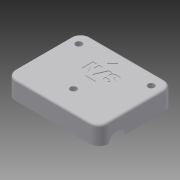
# Autodesk Inventor part: 137 V Dipole Top
Saved by Autodesk Inventor 2014 (Build 180170000, 170)
## iProperties
Created: 2023-07-11
Part Number: 137 V Dipole Top
Material: Generic
Document SubType Name: Modeling
Designer: VMUser
Density: 1 g/cm^3
Appearance: Default
Author: VMUser
Autodesk Inventor part; units mm, degrees
ref_plane "YZ Plane" through (0, 0, 0) normal (1, 0, 0) x (0, 1, 0)
sketch "Sketch1" plane through (0, 0, 0) normal (0, 1, 0) x (-1, 0, 0)
  line L0 (0, 0) -> (63.5, 0)
  line L1 (63.5, 0) -> (63.5, -50.8)
  line L2 (63.5, -50.8) -> (0, -50.8)
  line L3 (0, -50.8) -> (0, 0)
  line L4 (31.75, -50.8) -> (31.75, -30.48)
  line L5 (31.75, -30.48) -> (63.5, -12.1491)
  line L6 (31.75, -30.48) -> (0, -12.1491)
  line L7 (31.75, -30.48) -> (68.4117, -30.48) construction
  dimension "d0" = 63.5
  dimension "d1" = 50.8
  dimension "d2" = 20.32
  dimension "d3" = 120
  dimension "d4" = 150
  dimension "d5" = 120
  constraints: 16 end point, 3 parallel, 2 horizontal, 2 point on line, 1 equal length, 1 midpoint, 1 perpendicular
  measures "d0" distance of L1.end L2.end
  measures "d1" distance of L0.end L1.end
  measures "d2" distance of L4.start L4.end
  measures "d3" angle of L4 L5
  measures "d4" angle of L7 L6
  measures "d5" angle of L5 L6
extrude "Extrusion1" add sketch "Sketch1" along normal blind 12.7
ref_plane "Work Plane1" through (0, 0, 0) normal (0.8660254, 0, 0.5) x (0, 1, 0)
ref_plane "Work Plane2" through (-31.75, 0, -50.8) normal (-1, 0, 0) x (0, 0, 1)
sketch "Sketch2" plane through (0, 0, 0) normal (0.8660254, 0, 0.5) x (0, 1, 0)
  circle A0 centre (0, -10.5215) radius 4.826
  point P0 (0, 0)
  point P1 (0, -10.5215)
  dimension "d10" = 9.652
  constraints: 1 centre point, 1 coincident
  measures "d10" diameter of A0
extrude "Extrusion2" cut sketch "Sketch2" against normal up to surface surface through (-31.75, 0, -50.8) normal (-1, 0, 0)
mirror "Mirror2" about plane through (-31.75, 0, -50.8) normal (-1, 0, 0) of "Extrusion2"
sketch "Sketch5" plane through (0, 0, -50.8) normal (0, 0, -1) x (-1, 0, 0)
  circle A0 centre (31.75, 0) radius 3.556
  dimension "d18" = 7.112
  constraints: 1 centre point, 1 coincident
  measures "d18" diameter of A0
extrude "Extrusion4" cut sketch "Sketch5" against normal blind 20.32
sketch "Sketch6" plane through (0, 0, 0) normal (0, -1, 0) x (1, 0, 0)
  line L0 (-35.306, -33.9995) -> (-63.5, -17.7217) projected
  circle A0 centre (-60.2004, -19.6267) radius 1.3335
  line L1 (14.7857, -57.3474) -> (-82.6851, -1.0726) projected
  point P0 (0, 0)
  dimension "d21" = 2.667
  dimension "d23" = 1.905
  constraints: 1 centre point, 1 point on line
  measures "d21" diameter of A0
  measures "d23" vertical distance of L0.end A0.centre
revolve "Revolution1" cut sketch "Sketch6" angle 360 about axis through (-68.7607, 0, -9.1118) along (-0.8660254, 0, 0.5)
mirror "Mirror3" about plane through (-31.75, 0, -50.8) normal (-1, 0, 0) of "Revolution1"
sketch "Sketch11" plane through (0, 0, 0) normal (0, -1, 0) x (1, 0, 0)
  line L0 (-35.306, -50.8) -> (-35.306, -33.9995) projected
  circle A0 centre (-35.306, -42.3998) radius 1.016
  line L1 (-31.75, -60.96) -> (-31.75, 10.16) projected
  point P0 (0, 0)
  dimension "d33" = 2.032
  constraints: 1 centre point, 1 midpoint
  measures "d33" diameter of A0
revolve "Revolution4" cut sketch "Sketch11" angle 360 about axis through (-31.75, 0, -50.8) along (0, 0, 1)
sketch "Sketch12" plane through (0, 0, 0) normal (0, -1, 0) x (1, 0, 0)
  arc A0 (-6.9707, -10.6011) -> (-9.2804, -11.9346) centre (-8.1256, -11.2678) ccw projected
  arc A1 (-54.2196, -11.9346) -> (-56.5293, -10.6011) centre (-55.3744, -11.2678) ccw projected
  arc A2 (-9.3141, -10.6632) -> (-54.1859, -10.6632) centre (-31.75, -56.2403) ccw
  arc A3 (-9.4587, -11.3001) -> (-54.0413, -11.3001) centre (-31.75, -56.2403) ccw
  arc A4 (-8.881, -10.169) -> (-54.619, -10.169) centre (-31.75, -56.2403) ccw
  dimension "d35" = 50.8
  dimension "d36" = 0.635
  dimension "d37" = 0.635
  constraints: 12 point on circle, 3 centre point
  measures "d35" radius of A2
  measures "d36" radial gap between concentric circles of A4 A2
  measures "d37" radial gap between concentric circles of A2 A3
extrude "Extrusion5" cut sketch "Sketch12" against normal blind 1.27
sketch "Sketch13" plane through (0, 0, 0) normal (0, -1, 0) x (1, 0, 0)
  arc A0 (-35.306, -41.3838) -> (-35.306, -43.4158) centre (-35.306, -42.3998) ccw projected
  arc A1 (-61.3553, -18.96) -> (-59.0456, -20.2935) centre (-60.2004, -19.6267) ccw projected
  arc A2 (-59.8182, -20.9043) -> (-36.3024, -42.2011) centre (-29.5982, -11.167) ccw
  arc A3 (-60.4761, -20.9314) -> (-36.2063, -42.8707) centre (-29.5982, -11.167) ccw
  arc A4 (-59.2583, -20.5704) -> (-35.9624, -41.6242) centre (-29.5982, -11.167) ccw
  point P0 (0, 0)
  dimension "d40" = 31.75
  dimension "d41" = 0.635
  dimension "d42" = 0.635
  constraints: 12 point on circle, 3 centre point
  measures "d40" radius of A2
  measures "d41" radial gap between concentric circles of A4 A2
  measures "d42" radial gap between concentric circles of A2 A3
extrude "Extrusion6" cut sketch "Sketch13" against normal blind 1.27
mirror "Mirror4" about plane through (-31.75, 0, -50.8) normal (-1, 0, 0) of "Extrusion6"
sketch "Sketch14" plane through (0, 0, 0) normal (0, -1, 0) x (1, 0, 0)
  arc A0 (-35.9624, -41.6242) -> (-36.2063, -42.8707) centre (-35.306, -42.3998) ccw projected
  arc A1 (-27.2937, -42.8707) -> (-27.5376, -41.6242) centre (-28.194, -42.3998) ccw projected
  line L0 (-35.306, -42.3998) -> (-56.388, -42.3998) construction
  line L1 (-31.75, -34.2474) -> (-31.75, -30.48) construction
  point P0 (-31.75, -24.9074)
  point P1 (0, 0)
  point P2 (-31.75, -14.1124)
  point P3 (-7.112, -42.3998)
  dimension "d45" = 10.795
  dimension "d46" = 21.082
  constraints: 2 end point, 1 coincident, 1 horizontal, 1 symmetric about line
  measures "d45" distance of point (-31.75, -24.907) point (-31.75, -14.112)
  measures "d46" distance of L0.start L0.end
hole "Hole1" at (-31.75, 0, -14.1124) at (-56.388, 0, -42.3998) at (-7.112, 0, -42.3998) direction (0, 1, 0) diameter 4.3942 end through all counterbore diameter 10.287 counterbore depth 6.35
fillet "Fillet1" radius 6.35 4 edges at (-63.5, 6.35, -50.8) (0, 6.35, -50.8) (0, 6.35, 0) (-63.5, 6.35, 0)
sketch "Sketch15" plane through (0, 12.7, 0) normal (0, 1, 0) x (1, 0, 0)
  line L0 (-41.8086, 37.059) -> (-20.7861, 37.059) construction
  line L1 (-20.7861, 37.059) -> (-20.7861, 29.1175) construction
  line L2 (-20.7861, 29.1175) -> (-41.8086, 29.1175) construction
  line L3 (-41.8086, 29.1175) -> (-41.8086, 37.059) construction
  line L4 (-37.7464, 26.2268) -> (-25.2568, 26.2268) construction
  line L5 (-25.2568, 26.2268) -> (-25.2568, 22.3238) construction
  line L6 (-25.2568, 22.3238) -> (-37.7464, 22.3238) construction
  line L7 (-37.7464, 22.3238) -> (-37.7464, 26.2268) construction
  line L8 (-25.7536, 40.4291) -> (-38.2432, 40.4291) construction
  line L9 (-38.2432, 40.4291) -> (-38.2432, 44.3321) construction
  line L10 (-38.2432, 44.3321) -> (-25.7536, 44.3321) construction
  line L11 (-25.7536, 44.3321) -> (-25.7536, 40.4291) construction
  line L12 (-27.9889, 26.2268) -> (-31.8919, 22.3238)
  line L13 (-31.8919, 22.3238) -> (-35.7949, 26.2268)
  line L14 (-35.7949, 26.2268) -> (-27.9889, 26.2268)
  line L15 (-34.579, 36.8983) -> (-34.579, 29.2783)
  line L16 (-34.579, 29.2783) -> (-37.186, 29.2783)
  line L17 (-37.186, 29.2783) -> (-38.7307, 32.7408)
  line L18 (-38.7307, 32.7408) -> (-38.7307, 29.2783)
  line L19 (-38.7307, 29.2783) -> (-41.2171, 29.2783)
  line L20 (-41.2171, 29.2783) -> (-41.2171, 36.8983)
  line L21 (-41.2171, 36.8983) -> (-38.7307, 36.8983)
  line L22 (-38.7307, 36.8983) -> (-37.0654, 33.4644)
  line L23 (-37.0654, 33.4644) -> (-37.0654, 36.8983)
  line L24 (-37.0654, 36.8983) -> (-34.579, 36.8983)
  line L25 (-28.3429, 37.0476) -> (-31.7366, 29.1347)
  line L26 (-31.7366, 29.1347) -> (-33.8957, 29.1347)
  line L27 (-33.8957, 29.1347) -> (-30.479, 37.0476)
  line L28 (-30.479, 37.0476) -> (-28.3429, 37.0476)
  line L29 (-21.3718, 34.5956) -> (-24.1338, 34.5956)
  line L30 (-24.1338, 34.5956) -> (-24.1338, 35.1583)
  spline S0 degree 2 poles (-24.1338, 35.1583) (-24.1338, 35.5488) (-24.3463, 35.767) (-24.5932, 35.767) knots 0 0 0 1 2 2 2
  spline S1 degree 2 poles (-24.5932, 35.767) (-24.8631, 35.767) (-25.1387, 35.4742) (-25.1387, 35.1813) knots 0 0 0 1 2 2 2
  spline S2 degree 2 poles (-25.1387, 35.1813) (-25.1387, 34.8023) (-24.9837, 34.6128) knots 0 0 0 1 1 1
  spline S3 degree 2 poles (-24.9837, 34.6128) (-24.8286, 34.4176) (-24.1396, 34.142) knots 0 0 0 1 1 1
  spline S4 degree 2 poles (-24.1396, 34.142) (-22.1585, 33.3553) (-21.6417, 32.85) knots 0 0 0 1 1 1
  spline S5 degree 2 poles (-21.6417, 32.85) (-21.1249, 32.3446) (-21.1249, 31.2249) knots 0 0 0 1 1 1
  spline S6 degree 2 poles (-21.1249, 31.2249) (-21.1249, 30.4095) (-21.6991, 29.64) (-23.3356, 29.1175) (-24.4209, 29.1175) knots 0 0 0 1 2 3 3 3
  spline S7 degree 2 poles (-24.4209, 29.1175) (-25.6153, 29.1175) (-27.3036, 29.7204) (-27.8261, 30.6507) (-27.8261, 31.5063) knots 0 0 0 1 2 3 3 3
  line L31 (-27.8261, 31.5063) -> (-27.8261, 32.0058)
  line L32 (-27.8261, 32.0058) -> (-25.0641, 32.0058)
  line L33 (-25.0641, 32.0058) -> (-25.0641, 31.0813)
  spline S8 degree 2 poles (-25.0641, 31.0813) (-25.0641, 30.6564) (-24.8286, 30.4095) (-24.5358, 30.4095) knots 0 0 0 1 2 2 2
  spline S9 degree 2 poles (-24.5358, 30.4095) (-24.2372, 30.4095) (-23.9501, 30.7196) (-23.9501, 31.0239) knots 0 0 0 1 2 2 2
  spline S10 degree 2 poles (-23.9501, 31.0239) (-23.9501, 31.6958) (-24.2257, 31.9025) knots 0 0 0 1 1 1
  spline S11 degree 2 poles (-24.2257, 31.9025) (-24.5071, 32.1092) (-25.6153, 32.5973) knots 0 0 0 1 1 1
  spline S12 degree 2 poles (-25.6153, 32.5973) (-26.7236, 33.0854) (-27.4471, 33.5275) (-27.918, 34.3085) (-27.918, 34.9172) knots 0 0 0 1 2 3 3 3
  spline S13 degree 2 poles (-27.918, 34.9172) (-27.918, 35.7957) (-27.2461, 36.6054) (-25.7474, 37.059) (-24.6908, 37.059) knots 0 0 0 1 2 3 3 3
  spline S14 degree 2 poles (-24.6908, 37.059) (-23.5309, 37.059) (-21.9001, 36.5595) (-21.3718, 35.8015) (-21.3718, 34.8942) knots 0 0 0 1 2 3 3 3
  line L34 (-21.3718, 34.8942) -> (-21.3718, 34.5956)
  line L35 (-35.5111, 40.4291) -> (-31.6081, 44.3321)
  line L36 (-31.6081, 44.3321) -> (-27.7051, 40.4291)
  line L37 (-27.7051, 40.4291) -> (-35.5111, 40.4291)
  point P0 (0, 0)
  constraints: 6 other
emboss "Emboss1" sketch "Sketch15" operation cut depth 0.3969 direction (0, -1, 0)
fillet "Fillet2" radius 1.5875 8 edges at (-1.8599, 12.7, -1.8599) (0, 12.7, -25.4) (-1.8599, 12.7, -48.9401) (-31.75, 12.7, -50.8) (-61.6401, 12.7, -48.9401) (-63.5, 12.7, -25.4) (-61.6401, 12.7, -1.8599) (-31.75, 12.7, 0)
body "Solid1"
